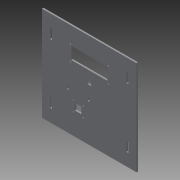
# Autodesk Inventor part: Tapa final
Saved by Autodesk Inventor 2014 (Build 180170000, 170)
## iProperties
Created: 2015-04-01
Part Number: Tapa final
Material: Genérico
Document SubType Name: Modeling
Designer: HP
Density: 1 g/cm^3
Appearance: Valor por defecto
Author: HP
Autodesk Inventor part; units mm, degrees
ref_plane "YZ Plane" through (0, 0, 0) normal (1, 0, 0) x (0, 1, 0)
ref_plane "XZ Plane" through (0, 0, 0) normal (0, 1, 0) x (-1, 0, 0)
ref_plane "XY Plane" through (0, 0, 0) normal (0, 0, 1) x (1, 0, 0)
sketch "Boceto1" plane through (0, 0, 0) normal (0, 1, 0) x (-1, 0, 0)
  line L0 (-105.368, 99.7227) -> (81.632, 99.7227)
  line L1 (81.632, 99.7227) -> (81.632, -87.2773)
  line L2 (81.632, -87.2773) -> (-105.368, -87.2773)
  line L3 (-105.368, -87.2773) -> (-105.368, 99.7227)
  line L4 (-89.368, 74.7227) -> (-85.368, 74.7227)
  line L5 (-85.368, 74.7227) -> (-85.368, 55.7227)
  line L6 (-85.368, 55.7227) -> (-89.368, 55.7227)
  line L7 (-89.368, 55.7227) -> (-89.368, 74.7227)
  line L8 (-89.368, -62.2773) -> (-85.368, -62.2773)
  line L9 (-85.368, -62.2773) -> (-85.368, -43.2773)
  line L10 (-85.368, -43.2773) -> (-89.368, -43.2773)
  line L11 (-89.368, -43.2773) -> (-89.368, -62.2773)
  line L12 (-47.368, 64.7227) -> (23.632, 64.7227)
  line L13 (23.632, 64.7227) -> (23.632, 40.7227)
  line L14 (23.632, 40.7227) -> (-47.368, 40.7227)
  line L15 (-47.368, 40.7227) -> (-47.368, 64.7227)
  circle A0 centre (-49.368, 67.7227) radius 1.5
  line L16 (-51.868, 70.2227) -> (28.132, 70.2227)
  line L17 (28.132, 70.2227) -> (28.132, 34.2227)
  line L18 (28.132, 34.2227) -> (-51.868, 34.2227)
  line L19 (-51.868, 34.2227) -> (-51.868, 70.2227)
  circle A1 centre (25.632, 67.7227) radius 1.5
  circle A2 centre (-49.368, 36.7227) radius 1.5
  circle A3 centre (25.632, 36.7227) radius 1.5
  line L20 (3.632, -29.2773) -> (16.632, -29.2773)
  line L21 (16.632, -29.2773) -> (16.632, -42.2773)
  line L22 (16.632, -42.2773) -> (3.632, -42.2773)
  line L23 (3.632, -42.2773) -> (3.632, -29.2773)
  line L24 (-11.968, -6.7773) -> (-8.468, -6.7773)
  line L25 (-8.468, -6.7773) -> (-8.468, -13.2773)
  line L26 (-8.468, -13.2773) -> (-11.968, -13.2773)
  line L27 (-11.968, -13.2773) -> (-11.968, -6.7773)
  line L28 (32.232, -6.7773) -> (28.732, -6.7773)
  line L29 (28.732, -6.7773) -> (28.732, -13.2773)
  line L30 (28.732, -13.2773) -> (32.232, -13.2773)
  line L31 (32.232, -13.2773) -> (32.232, -6.7773)
  line L32 (65.632, 74.7227) -> (61.632, 74.7227)
  line L33 (61.632, 74.7227) -> (61.632, 55.7227)
  line L34 (61.632, 55.7227) -> (65.632, 55.7227)
  line L35 (65.632, 55.7227) -> (65.632, 74.7227)
  line L36 (65.632, -43.2773) -> (65.632, -62.2773)
  line L37 (65.632, -62.2773) -> (61.632, -62.2773)
  line L38 (61.632, -62.2773) -> (61.632, -43.2773)
  line L39 (61.632, -43.2773) -> (65.632, -43.2773)
  point P0 (0, 0)
  dimension "d0" = 187
  dimension "d1" = 187
  dimension "d2" = 16
  dimension "d3" = 25
  dimension "d4" = 19
  dimension "d5" = 4
  dimension "d7" = 71
  dimension "d8" = 58
  dimension "d10" = 3
  dimension "d11" = 36
  dimension "d12" = 80
  dimension "d13" = 4.5
  dimension "d14" = 5.5
  dimension "d15" = 2.5
  dimension "d16" = 2.5
  dimension "d17" = 35
  dimension "d26" = 16
  dimension "d27" = 25
  dimension "d28" = 4
  dimension "d29" = 19
  dimension "d30" = 2.5
  dimension "d31" = 2.5
  dimension "d32" = 2.5
  dimension "d33" = 2.5
  dimension "d34" = 2.5
  dimension "d35" = 2.5
  dimension "d36" = 13
  dimension "d37" = 13
  dimension "d38" = 65
  dimension "d39" = 45
  dimension "d40" = 6.5
  dimension "d41" = 3.5
  dimension "d42" = 29
  dimension "d45" = 29
  dimension "d46" = 3.5
  dimension "d47" = 6.5
  dimension "d48" = 16
  dimension "d49" = 19
  dimension "d50" = 4
  dimension "d51" = 25
  dimension "d52" = 16
  dimension "d53" = 4
  dimension "d54" = 19
  dimension "d55" = 25
  dimension "d72" = 37.2
  dimension "d73" = 12.1
  dimension "d74" = 24
  constraints: 80 end point, 12 parallel, 6 horizontal, 6 perpendicular, 4 centre point
  measures "d0" distance of L0.start L0.end
  measures "d1" distance of L0.end L1.end
  measures "d2" distance between parallel lines of L3 L7
  measures "d3" distance between parallel lines of L0 L4
  measures "d4" distance between parallel lines of L6 L4
  measures "d5" distance between parallel lines of L5 L7
  measures "d7" distance between parallel lines of L13 L15
  measures "d8" distance between parallel lines of L3 L15
  measures "d10" diameter of A0
  measures "d11" distance between parallel lines of L18 L16
  measures "d12" distance between parallel lines of L17 L19
  measures "d13" distance between parallel lines of L17 L13
  measures "d14" distance between parallel lines of L16 L12
  measures "d15" distance from line of L19 A0.centre
  measures "d16" distance from line of L16 A0.centre
  measures "d17" distance between parallel lines of L0 L12
  measures "d26" distance between parallel lines of L3 L11
  measures "d27" distance from line of L2 L8.end
  measures "d28" distance between parallel lines of L9 L11
  measures "d29" distance of L8.end L9.end
  measures "d30" distance from line of L16 A1.centre
  measures "d31" distance from line of L17 A1.centre
  measures "d32" distance from line of L17 A3.centre
  measures "d33" distance from line of L18 A3.centre
  measures "d34" distance from line of L19 A2.centre
  measures "d35" distance from line of L18 A2.centre
  measures "d36" distance of L20.end L21.end
  measures "d37" distance between parallel lines of L21 L23
  measures "d38" distance between parallel lines of L1 L21
  measures "d39" distance between parallel lines of L2 L22
  measures "d40" distance of L24.end L25.end
  measures "d41" distance between parallel lines of L25 L27
  measures "d42" distance between parallel lines of L22 L26
  measures "d45" distance between parallel lines of L30 L22
  measures "d46" distance between parallel lines of L31 L29
  measures "d47" distance between parallel lines of L30 L28
  measures "d48" distance between parallel lines of L1 L35
  measures "d49" distance between parallel lines of L32 L34
  measures "d50" distance between parallel lines of L33 L35
  measures "d51" distance between parallel lines of L0 L32
  measures "d52" distance between parallel lines of L1 L36
  measures "d53" distance between parallel lines of L36 L38
  measures "d54" distance between parallel lines of L37 L39
  measures "d55" distance between parallel lines of L2 L37
  measures "d72" distance between parallel lines of L29 L25
  measures "d73" distance between parallel lines of L25 L23
  measures "d74" distance between parallel lines of L14 L12
extrude "Extrusión1" add sketch "Boceto1" along normal blind 3 contours L0 L1 L2 L3 | L16 L17 L18 L19
sketch "Boceto2" plane through (0, 3, 0) normal (0, 1, 0) x (1, 0, 0)
  line L0 (-16.632, 29.2773) -> (-16.632, 42.2773) projected
  line L1 (-16.632, 42.2773) -> (-3.632, 42.2773) projected
  line L2 (-3.632, 42.2773) -> (-3.632, 29.2773) projected
  line L3 (-3.632, 29.2773) -> (-16.632, 29.2773) projected
  line L4 (3.368, 22.2773) -> (-23.632, 22.2773)
  line L5 (-23.632, 22.2773) -> (-23.632, 49.2773)
  line L6 (-23.632, 49.2773) -> (3.368, 49.2773)
  line L7 (3.368, 49.2773) -> (3.368, 22.2773)
  circle A0 centre (-0.132, 25.7773) radius 1.5
  line L8 (-10.132, 22.2773) -> (-10.132, 49.2773)
  line L9 (3.368, 35.7773) -> (-23.632, 35.7773)
  circle A1 centre (-20.132, 25.7773) radius 1.5
  circle A2 centre (-0.132, 45.7773) radius 1.5
  circle A3 centre (-20.132, 45.7773) radius 1.5
  point P0 (0, 0)
  dimension "d58" = 7
  dimension "d59" = 7
  dimension "d60" = 7
  dimension "d61" = 7
  dimension "d62" = 3
  dimension "d63" = 3.5
  dimension "d64" = 3.5
  dimension "d75" = 3.5
  constraints: 12 end point, 4 centre point, 4 midpoint, 3 symmetric about line, 2 parallel, 1 horizontal, 1 perpendicular, 3 other
  measures "d58" distance between parallel lines of L4 L3
  measures "d59" distance between parallel lines of L5 L0
  measures "d60" distance between parallel lines of L6 L1
  measures "d61" distance between parallel lines of L7 L2
  measures "d62" diameter of A0
  measures "d63" distance from line of L7 A0.centre
  measures "d64" distance from line of A0.centre L4
  measures "d75" distance from line of L5 A1.centre
extrude "Extrusión2" cut sketch "Boceto2" against normal through all contours A0 | A1 | A2 | A3
sketch "Boceto3" plane through (0, 3, 0) normal (0, 1, 0) x (1, 0, 0)
  line L0 (-81.632, -99.7227) -> (105.368, -99.7227) projected
  line L1 (-81.632, 87.2773) -> (-81.632, -99.7227) projected
  circle A0 centre (11.868, -19.7227) radius 4.75
  point P0 (0, 0)
  dimension "d67" = 9.5
  dimension "d68" = 93.5
  dimension "d69" = 80
  constraints: 1 centre point
  measures "d67" diameter of A0
  measures "d68" distance from line of L1 A0.centre
  measures "d69" distance from line of L0 A0.centre
extrude "Extrusión3" cut sketch "Boceto3" against normal through all
